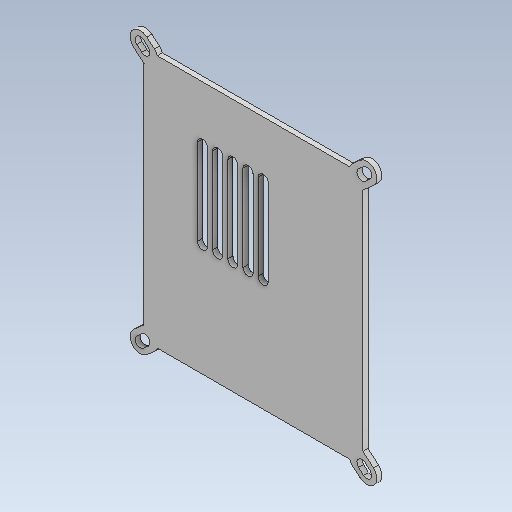
# Autodesk Inventor part: Case Cover Rev D
Saved by Autodesk Inventor 2021 (Build 250183000, 183)
## iProperties
Created: 2021-07-31
Part Number: Case Cover Rev D
Material: Generic
Document SubType Name: Modeling
Designer: cmzgt
Density: 1 g/cm^3
Appearance: Default
Author: cmzgt
Autodesk Inventor part; units mm, degrees
ref_plane "YZ Plane" through (0, 0, 0) normal (1, 0, 0) x (0, 1, 0)
ref_plane "XZ Plane" through (0, 0, 0) normal (0, 1, 0) x (-1, 0, 0)
ref_plane "XY Plane" through (0, 0, 0) normal (0, 0, 1) x (1, 0, 0)
sketch "Sketch1" plane through (0, 0, 0) normal (0, 0, 1) x (1, 0, 0)
  circle A0 centre (44.8094, -51.3621) radius 1.975 projected
  circle A1 centre (-44.8094, -51.3621) radius 1.975 projected
  circle A2 centre (-44.8094, 51.3621) radius 1.975 projected
  circle A3 centre (44.8094, 51.3621) radius 1.975 projected
  line L0 (38.0119, 50.05) -> (-38.0119, 50.05) projected
  arc A4 (-38.0119, 50.05) -> (-39.1663, 51.7567) centre (-41.7906, 48.7379) ccw projected
  line L1 (-42.1852, 54.381) -> (-39.1663, 51.7567) projected
  arc A5 (-42.1852, 54.381) -> (-47.4337, 48.3433) centre (-44.8094, 51.3621) ccw projected
  line L2 (-43.3, 44.7499) -> (-47.4337, 48.3433) projected
  line L3 (-43.3, 44.7499) -> (-43.3, -44.7499) projected
  line L4 (-47.4337, -48.3433) -> (-43.3, -44.7499) projected
  arc A6 (-47.4337, -48.3433) -> (-42.1852, -54.381) centre (-44.8094, -51.3621) ccw projected
  line L5 (-39.1663, -51.7567) -> (-42.1852, -54.381) projected
  arc A7 (-39.1663, -51.7567) -> (-38.0119, -50.05) centre (-41.7906, -48.7379) ccw projected
  line L6 (-38.0119, -50.05) -> (38.0119, -50.05) projected
  arc A8 (38.0119, -50.05) -> (39.1663, -51.7567) centre (41.7906, -48.7379) ccw projected
  line L7 (42.1852, -54.381) -> (39.1663, -51.7567) projected
  arc A9 (42.1852, -54.381) -> (47.4337, -48.3433) centre (44.8094, -51.3621) ccw projected
  line L8 (43.3, -44.7499) -> (47.4337, -48.3433) projected
  line L9 (43.3, -44.7499) -> (43.3, 44.7499) projected
  line L10 (47.4337, 48.3433) -> (43.3, 44.7499) projected
  arc A10 (47.4337, 48.3433) -> (42.1852, 54.381) centre (44.8094, 51.3621) ccw projected
  line L11 (39.1663, 51.7567) -> (42.1852, 54.381) projected
  arc A11 (39.1663, 51.7567) -> (38.0119, 50.05) centre (41.7906, 48.7379) ccw projected
  line L12 (-40.1, -44.85) -> (-40.1, 44.85) projected
  arc A12 (-38.1, 46.85) -> (-40.1, 44.85) centre (-38.1, 44.85) ccw projected
  line L13 (-38.1, 46.85) -> (38.1, 46.85) projected
  arc A13 (40.1, 44.85) -> (38.1, 46.85) centre (38.1, 44.85) ccw projected
  line L14 (40.1, 44.85) -> (40.1, -44.85) projected
  arc A14 (38.1, -46.85) -> (40.1, -44.85) centre (38.1, -44.85) ccw projected
  line L15 (38.1, -46.85) -> (-38.1, -46.85) projected
  arc A15 (-40.1, -44.85) -> (-38.1, -46.85) centre (-38.1, -44.85) ccw projected
  point P0 (0, 0)
extrude "Extrusion1" add sketch "Sketch1" along normal blind 2 contours A11 L11 A10 L10 L9 L8 A9 L7 A8 L6 A7 L5 A6 L4 L3 L2 A5 L1 A4 L0 | L12 A12 L13 A13 L14 A14 L15 A15
sketch "Sketch2" plane through (0, 0, 2) normal (0, 0, 1) x (1, 0, 0)
  circle A0 centre (-44.8094, 51.3621) radius 1.975 projected
  circle A1 centre (-44.8094, -51.3621) radius 1.975 projected
  circle A2 centre (44.8094, -51.3621) radius 1.975 projected
  circle A3 centre (44.8094, 51.3621) radius 1.975 projected
  circle A4 centre (44.8094, 51.3621) radius 1.975 construction
  line L0 (44.8094, 51.3621) -> (42.8472, 49.6564) construction
  line L1 (43.5137, 52.8527) -> (41.5515, 51.1469)
  line L2 (44.1429, 48.1658) -> (46.1051, 49.8716)
  arc A5 (46.1051, 49.8716) -> (43.5137, 52.8527) centre (44.8094, 51.3621) ccw
  arc A6 (41.5515, 51.1469) -> (44.1429, 48.1658) centre (42.8472, 49.6564) ccw
  line L3 (43.3, -44.7499) -> (43.3, 44.7499) projected
  line L4 (43.3, 0) -> (-43.3, 0) construction
  line L5 (-43.3, 44.7499) -> (-43.3, -44.7499) construction
  line L6 (38.0119, 50.05) -> (-38.0119, 50.05) construction
  line L7 (0, 50.05) -> (0, -50.05) construction
  line L8 (-38.0119, -50.05) -> (38.0119, -50.05) construction
  line L9 (43.5137, -52.8527) -> (41.5515, -51.1469)
  line L10 (44.1429, -48.1658) -> (46.1051, -49.8716)
  arc A7 (44.1429, -48.1658) -> (41.5515, -51.1469) centre (42.8472, -49.6564) ccw
  line L11 (-43.5137, 52.8527) -> (-41.5515, 51.1469)
  line L12 (-44.1429, 48.1658) -> (-46.1051, 49.8716)
  arc A8 (-44.1429, 48.1658) -> (-41.5515, 51.1469) centre (-42.8472, 49.6564) ccw
  line L13 (-44.1429, -48.1658) -> (-46.1051, -49.8716)
  arc A9 (-41.5515, -51.1469) -> (-44.1429, -48.1658) centre (-42.8472, -49.6564) ccw
  line L14 (-43.5137, -52.8527) -> (-41.5515, -51.1469)
  point P0 (0, 0)
  point P1 (43.8283, 50.5092)
  point P2 (46.1051, 49.8716)
  point P3 (-43.5137, 52.8527)
  point P4 (-46.1051, 49.8716)
  point P5 (-46.1051, -49.8716)
  point P6 (-43.5137, -52.8527)
  point P7 (43.5137, -52.8527)
  point P8 (46.1051, -49.8716)
  dimension "d4" = 1.3
  dimension "d5" = 131
  constraints: 24 end point, 15 symmetric about line, 10 point on circle, 5 centre point, 5 midpoint, 5 tangent, 1 parallel, 3 other
  measures "d4" distance of A3.centre point (43.828, 50.509)
  measures "d5" angle of L3 L2
extrude "Extrusion2" cut sketch "Sketch2" against normal up to surface (2 mm away) contours A0 L11 A8 L12 | A1 L13 A9 L14 | A2 L9 A7 L10 | A3 | A3 L2 A6 L1
sketch "Sketch3" plane through (0, 0, 2) normal (0, 0, 1) x (1, 0, 0)
  line L0 (-15.2986, 18.4674) -> (-1.1867, 18.4674) projected
  line L1 (-1.1867, 18.4674) -> (-1.1867, 4.4942) projected
  line L2 (-1.1867, 4.4942) -> (-15.2986, 4.4942) projected
  line L3 (-15.2986, 4.4942) -> (-15.2986, 18.4674) projected
  line L4 (-8.1427, -5.5192) -> (-8.1427, 28.4808) construction
  line L5 (-6.1427, -5.5192) -> (-6.1427, 28.4808)
  line L6 (-10.1427, 28.4808) -> (-10.1427, -5.5192)
  arc A0 (-10.1427, -5.5192) -> (-6.1427, -5.5192) centre (-8.1427, -5.5192) ccw
  arc A1 (-6.1427, 28.4808) -> (-10.1427, 28.4808) centre (-8.1427, 28.4808) ccw
  arc A2 (-0.1427, 28.4808) -> (-4.1427, 28.4808) centre (-2.1427, 28.4808) ccw
  line L7 (-0.1427, -5.5192) -> (-0.1427, 28.4808)
  line L8 (-4.1427, 28.4808) -> (-4.1427, -5.5192)
  arc A3 (-4.1427, -5.5192) -> (-0.1427, -5.5192) centre (-2.1427, -5.5192) ccw
  line L9 (5.8573, -5.5192) -> (5.8573, 28.4808)
  arc A4 (5.8573, 28.4808) -> (1.8573, 28.4808) centre (3.8573, 28.4808) ccw
  line L10 (1.8573, 28.4808) -> (1.8573, -5.5192)
  arc A5 (1.8573, -5.5192) -> (5.8573, -5.5192) centre (3.8573, -5.5192) ccw
  line L11 (-16.1427, 28.4808) -> (-16.1427, -5.5192)
  arc A6 (-12.1427, 28.4808) -> (-16.1427, 28.4808) centre (-14.1427, 28.4808) ccw
  line L12 (-12.1427, -5.5192) -> (-12.1427, 28.4808)
  arc A7 (-16.1427, -5.5192) -> (-12.1427, -5.5192) centre (-14.1427, -5.5192) ccw
  line L13 (-22.1427, 28.4808) -> (-22.1427, -5.5192)
  arc A8 (-18.1427, 28.4808) -> (-22.1427, 28.4808) centre (-20.1427, 28.4808) ccw
  line L14 (-18.1427, -5.5192) -> (-18.1427, 28.4808)
  arc A9 (-22.1427, -5.5192) -> (-18.1427, -5.5192) centre (-20.1427, -5.5192) ccw
  point P0 (0, 0)
  point P1 (-8.1427, 11.4808)
  dimension "d8" = 17
  dimension "d9" = 4
  dimension "d12" = 6
  dimension "d19" = 6
  dimension "d26" = 6
  constraints: 24 end point, 20 point on circle, 10 centre point, 4 tangent, 3 horizontal, 1 midpoint, 1 parallel, 1 vertical, 40 other
  measures "d8" distance of point (-8.143, 11.481) L4.end
  measures "d9" diameter of A1
  measures "d12" distance of L4.end A2.centre
  measures "d19" distance of L7.start L9.start
  measures "d26" distance of L6.start L11.start
extrude "Extrusion3" cut sketch "Sketch3" against normal up to surface (2 mm away) contours L3 L2 L12 A7 L11 A6 L0 | L0 L12 L2 L3 | L6 A1 L5 L0 | L0 L5 L2 L6 | L2 L5 A0 L6 | L8 A2 L7 A3 L2 L1 L0 | L0 L1 L2 L8 | A5 L10 A4 L9 | A8 L14 A9 L13
body "Solid1"
